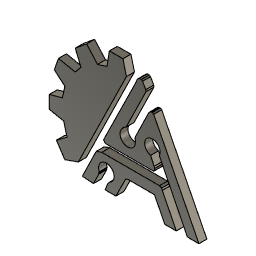
Logo_Ares_2 v4 (Autodesk Fusion 360 archive; units mm, degrees)
design "Logo_Ares_seul"
Autodesk Fusion 360 part; units mm, degrees
sketch "Esquisse3" plane through (0, 2, 0) normal (0, 1, 0) x (-1, 0, 0)
  line L0 (0, 25) -> (-24, 25)
  line L1 (-24, 25) -> (-24, 0)
  line L2 (-24, 0) -> (0, 0)
  line L3 (0, 0) -> (0, 25)
  line L4 (-21.448, 5.4824) -> (-20, 5.4824)
  line L5 (-20, 5.4824) -> (-16.5487, 12.4198)
  circle A0 centre (-15.6, 13) radius 0.9683
  circle A1 centre (-12.5, 12.5) radius 0.9713
  circle A2 centre (-9.8142, 7.4586) radius 0.9789
  line L6 (-15.3731, 12.0586) -> (-15.7623, 11.2146)
  line L7 (-15.7623, 11.2146) -> (-15.8189, 11.0919)
  line L8 (-15.8189, 11.0919) -> (-15.8811, 10.8807)
  line L9 (-15.8811, 10.8807) -> (-15.8811, 10.6756)
  line L10 (-15.8811, 10.6756) -> (-15.8811, 10.6405)
  line L11 (-15.8811, 10.6405) -> (-15.7272, 10.5109)
  line L12 (-15.7272, 10.5109) -> (-9.9, 10.5109)
  line L13 (-9.9, 10.5109) -> (-9.7, 10.5109)
  line L14 (-9.7, 10.5109) -> (-9.4749, 10.7781)
  line L15 (-9.4749, 10.7781) -> (-9.5875, 11.0568)
  line L16 (-9.5875, 11.0568) -> (-13.5, 19)
  line L17 (-13.5, 19) -> (-13.7093, 19.5183)
  line L18 (-13.7093, 19.5183) -> (-13.9534, 19.7239)
  line L19 (-13.9534, 19.7239) -> (-14.2, 19.7239)
  line L20 (-14.2, 19.7239) -> (-14.3641, 19.6211)
  line L21 (-14.3641, 19.6211) -> (-14.5703, 19.2561)
  line L22 (-14.5703, 19.2561) -> (-14.7167, 18.9969)
  line L23 (-14.7167, 18.9969) -> (-14.7682, 18.9058)
  line L24 (-14.7682, 18.9058) -> (-14.8, 18.7)
  line L25 (-14.8, 18.7) -> (-12.3, 13.6)
  line L26 (-12.3, 13.6) -> (-11.9733, 13.4155)
  line L27 (-11.9733, 13.4155) -> (-11.7239, 13.0839)
  line L28 (-21.448, 5.4824) -> (-15.7676, 16.7212)
  line L29 (-15.7676, 16.7212) -> (-15.6, 16.8425)
  line L30 (-15.6, 16.8425) -> (-15.5, 16.8425)
  line L31 (-15.5, 16.8425) -> (-15.4271, 16.8056)
  line L32 (-15.4271, 16.8056) -> (-15.2601, 16.7212)
  line L33 (-15.2601, 16.7212) -> (-15.1097, 16.5133)
  line L34 (-15.1097, 16.5133) -> (-13.5, 13.2)
  line L35 (-13.5, 13.2) -> (-13.4125, 13.0199)
  line L36 (-13.4125, 13.0199) -> (-13.4125, 12.8327)
  line L37 (-13.4344, 12.7651) -> (-13.4125, 12.9263)
  line L38 (-16.5487, 12.4198) -> (-16.4708, 12.5764)
  line L39 (-18.6078, 5.4476) -> (-17.1615, 5.4476)
  line L40 (-17.1615, 5.4476) -> (-15.8607, 8.0212)
  line L41 (-15.8607, 8.0212) -> (-12.5, 8.0212)
  line L42 (-12.5, 8.0212) -> (-12.2305, 7.885)
  line L43 (-12.2305, 7.885) -> (-11.0177, 5.4476)
  line L44 (-11.0177, 5.4476) -> (-9.6577, 5.4476)
  line L45 (-9.6577, 5.4476) -> (-10, 6.3)
  line L46 (-10, 6.3) -> (-10.2242, 6.5696)
  line L47 (-8.923, 7.0537) -> (-8.8514, 6.8754)
  line L48 (-8.8514, 6.8754) -> (-8.8872, 6.7833)
  line L49 (-8.8872, 6.7833) -> (-8.2, 5.4)
  line L50 (-8.2, 5.4) -> (-6.8, 5.5)
  line L51 (-6.8, 5.5) -> (-8.5436, 9.0762)
  line L52 (-8.5436, 9.0762) -> (-8.9, 9.2)
  line L53 (-8.9, 9.2) -> (-9.2369, 9.317)
  line L54 (-9.2369, 9.317) -> (-16.5, 9.317)
  line L55 (-16.5, 9.317) -> (-16.6325, 9.2585)
  line L56 (-16.6325, 9.2585) -> (-16.7698, 9.1979)
  line L57 (-16.7698, 9.1979) -> (-16.8443, 8.9836)
  line L58 (-16.8443, 8.9836) -> (-18.6078, 5.4476)
  line L59 (-11.9031, 20.8338) -> (-10.1917, 20.8338)
  line L60 (-10.1917, 20.8338) -> (-9.9, 18.9972)
  line L61 (-9.9, 18.9972) -> (-8.7099, 18.6215)
  line L62 (-8.7099, 18.6215) -> (-7.3324, 20.1659)
  line L63 (-7.3324, 20.1659) -> (-5.9132, 18.9972)
  line L64 (-5.9132, 18.9972) -> (-6.6228, 17.2649)
  line L65 (-6.6228, 17.2649) -> (-5.9132, 16.3883)
  line L66 (-5.9132, 16.3883) -> (-3.8053, 16.8266)
  line L67 (-3.8053, 16.8266) -> (-3.2835, 15.3239)
  line L68 (-3.2835, 15.3239) -> (-4.5983, 14.1969)
  line L69 (-4.5983, 14.1969) -> (-4.3044, 12.7832)
  line L70 (-4.3044, 12.7832) -> (-2.6365, 12.3186)
  line L71 (-2.6365, 12.3186) -> (-2.6365, 10.7115)
  line L72 (-2.6365, 10.7115) -> (-4.4514, 10.3342)
  line L73 (-4.4514, 10.3342) -> (-4.8795, 8.7976)
  line L74 (-4.8795, 8.7976) -> (-3.5439, 7.7896)
  line L75 (-3.5439, 7.7896) -> (-4.6, 6.2)
  line L76 (-4.6, 6.2) -> (-6.3, 6.8)
  line L77 (-6.3, 6.8) -> (-12.3438, 19.1111)
  line L78 (-12.3438, 19.1111) -> (-11.9031, 20.8338)
  constraint horizontal L4
  constraint coincident A0 L6.start
  constraint parallel L6 L7
  constraint vertical L9
  constraint perpendicular L9 L12
  constraint perpendicular L9 L13
  constraint perpendicular L11 L14
  constraint parallel L15 L17
  constraint perpendicular L14 L18
  constraint horizontal L19
  constraint parallel L21 L22
  constraint perpendicular L21 L26
  constraint coincident A1 L27.end
  constraint tangent A1 L27
  constraint parallel L4 L30
  constraint perpendicular L28 L31
  constraint parallel L31 L32
  constraint perpendicular L29 L33
  constraint coincident A1 L36.end
  constraint vertical L36
  constraint coincident A1 L37.start
  constraint midpoint L36 L37.end
  constraint coincident A0 L38.end
  constraint parallel L5 L38
  constraint horizontal L39
  constraint parallel L28 L40
  constraint parallel L39 L41
  constraint perpendicular L40 L42
  constraint parallel L41 L44
  constraint coincident A2 L46.end
  constraint coincident A2 L47.start
  constraint parallel L45 L47
  constraint parallel L52 L53
  constraint horizontal L54
  constraint parallel L55 L56
  constraint perpendicular L53 L57
  constraint parallel L13 L59
  constraint perpendicular L66 L69
  constraint vertical L71
  constraint perpendicular L69 L72
  constraint perpendicular L70 L73
extrude "Extrusion2" add sketch "Esquisse3" along normal blind 1 contours L4 L5 A0 A1 L6 L7 L8 L9 L10 L11 L12 L13 L14 L15 L16 L17 L18 L19 L20 L21 L22 L23 L24 L25 L26 L27 L28 L29 L30 L31 L32 L33 L34 L35 L36 L37 L38 | A2 L39 L40 L41 L42 L43 L44 L45 L46 L47 L48 L49 L50 L51 L52 L53 L54 L55 L56 L57 L58 | L59 L60 L61 L62 L63 L64 L65 L66 L67 L68 L69 L70 L71 L72 L73 L74 L75 L76 L77 L78 makes body 1 at (13.5333, 2, 17.1) makes body 2 at (8.1857, 2, 14.0998) makes body 3 at (12.7456, 2, 8.8851)
